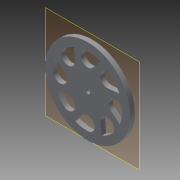
# Autodesk Inventor part: hubSpider
Saved by Autodesk Inventor 2013 (Build 170138000, 138)
## iProperties
Created: 2013-01-20
Part Number: hubSpider
Material: Generic
Document SubType Name: Modeling
Designer: Nano
Density: 1 g/cm^3
Author: Nano
Autodesk Inventor part; units mm, degrees
ref_plane "YZ Plane" through (0, 0, 0) normal (1, 0, 0) x (0, 1, 0)
ref_plane "XZ Plane" through (0, 0, 0) normal (0, 1, 0) x (-1, 0, 0)
ref_plane "XY Plane" through (0, 0, 0) normal (0, 0, 1) x (1, 0, 0)
ref_plane "Work Plane1" through (0, 0, 0) normal (0, 0, 1) x (1, 0, 0)
sketch "Sketch1" plane through (0, 0, 0) normal (0, 0, 1) x (1, 0, 0)
  circle A0 centre (0, 0) radius 117.475 projected
  point P0 (0, 0)
extrude "Extrusion1" add sketch "Sketch1" along normal blind 12.7
sketch "Sketch3" plane through (0, 0, 12.7) normal (0, 0, 1) x (1, 0, 0)
  circle A0 centre (0, 0) radius 117.475 projected
  circle A1 centre (0, 0) radius 6.35
  circle A2 centre (0, 0) radius 95.25 projected
  circle A3 centre (0, 76.2) radius 19.05
  line L0 (34.6081, 88.7403) -> (14.8223, 64.2332)
  point P0 (0, 95.25)
  dimension "d15" = 12.7
  dimension "d16" = 38.1
  constraints: 4 point on circle, 2 centre point, 2 coincident, 2 end point, 2 tangent
  measures "d15" diameter of A1
  measures "d16" diameter of A3
extrude "Extrusion5" cut sketch "Sketch3" against normal through all contours A1 | L0 A3 A2 | A3 picked at (25.5173, 87.1725)
pattern_circular "Circular Pattern2" count 8 over 360 about axis through (0, 0, 12.7) along (0, 0, -1) of "Extrusion5"
body "Solid1"
